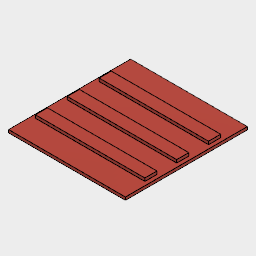
HDD Base Plate v5 (Autodesk Fusion 360 design; units mm, degrees)
Autodesk Fusion 360 part; units mm, degrees
sketch "Sketch1" plane through (0, 0, 0) normal (0, 1, 0) x (1, 0, 0) in component "HDD"
  line L0 (0, 0) -> (-146, 0)
  line L1 (-146, 0) -> (-146, 25.4)
  line L2 (-146, 25.4) -> (0, 25.4)
  line L3 (0, 25.4) -> (0, 0)
  dimension "d1" = 146
  dimension "d2" = 25.4
  measures "d1" distance of L0.start L0.end
  measures "d2" distance of L0.start L2.end
extrude "Extrude1" add sketch "Sketch1" along normal blind 101.6 makes body 1 in component "HDD"
sketch "Sketch1 (2)" plane through (0, 0, 0) normal (0, 1, 0) x (1, 0, 0) in component "Base"
  line L0 (0, 0) -> (-146, 0)
  line L1 (-146, 0) -> (-146, 153)
  line L2 (-146, 153) -> (0, 153)
  line L3 (0, 153) -> (0, 0)
  dimension "d8" = 153
  dimension "d9" = 146
  measures "d8" distance of L0.start L2.end
  measures "d9" distance of L0.start L0.end
extrude "Extrude1'" add sketch "Sketch1 (2)" along normal blind 4 separate body makes body 2 in component "Base"
pattern_linear "R-Pattern1" [suppressed]
extrude "Extrude2" add 1 faces at (-48.6667, 1.3333, 0) along direction (0, 0, 1) blind 5 on bodies 2 bodies 2 in component "Base"
extrude "Extrude3" add 1 faces at (0, 2.6667, -100.3333) along direction (1, 0, 0) blind 5 on bodies 2 bodies 2 in component "Base"
extrude "Extrude4" add 1 faces at (-95.6667, 1.3333, -153) along direction (0, 0, -1) blind 5 on bodies 2 bodies 2 in component "Base"
extrude "Extrude5" add 1 faces at (-146, 2.6667, -103.6667) along direction (-1, 0, 0) blind 5 on bodies 2 bodies 2 in component "Base"
sketch "Sketch1 (3)" plane through (0, 0, -127.6) normal (0, 0, 1) x (1, 0, 0)
  line L0 (-146, 0) -> (0, 0)
  line L1 (0, 0) -> (0, 101.6)
  line L2 (0, 101.6) -> (-146, 101.6)
  line L3 (-146, 101.6) -> (-146, 0)
sketch "Sketch2" plane through (0, 4, 0) normal (0, 1, 0) x (-1, 0, 0)
  line L0 (151, 5) -> (-5, 5)
  line L1 (-5, 5) -> (-5, -158)
  line L2 (-5, -158) -> (151, -158)
  line L3 (151, -158) -> (151, 5)
sketch "Sketch3" plane through (0, 0, 0) normal (0, 1, 0) x (1, 0, 0)
  line L0 (-146, 127.6) -> (0, 127.6)
  line L1 (0, 127.6) -> (0, 110.4667)
  line L2 (0, 110.4667) -> (-146, 110.4667)
  line L3 (-146, 110.4667) -> (-146, 127.6)
  point P0 (-146, 127.6)
  point P1 (0, 110.4667)
extrude "Extrude1''" add sketch "Sketch3" along normal blind 4 separate body makes body 3
move_body "Move1" bodies 3 to x (1, 0, 0) y (0, 1, 0) z (0, 0, 1) at (0, 35, 0)
extrude "Extrude2'" cut 1 faces at (-48.6667, 36.3333, -110.4667) along direction (0, 0, -1) blind 0.5 on bodies 3 bodies 3
extrude "Extrude3'" cut 1 faces at (-97.3333, 36.3333, -127.6) along direction (0, 0, 1) blind 0.5 on bodies 3 bodies 3
move_body "Align1" bodies 3 to x (1, 0, 0) y (0, 1, 0) z (0, 0, 1) at (0, -31, 0)
pattern_linear "R-Pattern1'" count 3 spacing 42.5 along (0, 0, 1) of bodies 3 makes body 4 at (-97.3333, 4, -79.2222) makes body 5 at (-97.3333, 4, -36.7222)
combine "Combine1" operation add target body 4 tool bodies 5 3 2
component "HDD" placed x (1, 0, 0) y (0, 1, 0) z (0, 0, 1) at (0, 0, 0)
component "Base" placed x (1, 0, 0) y (0, 1, 0) z (0, 0, 1) at (0, 0, 0)
component "HDD" placed x (1, 0, 0) y (0, 1, 0) z (0, 0, 1) at (0, 0, -42.5333)
component "HDD" placed x (1, 0, 0) y (0, 1, 0) z (0, 0, 1) at (0, 0, -85.0667)
component "HDD" placed x (1, 0, 0) y (0, 1, 0) z (0, 0, 1) at (0, 0, -127.6)
equation "d1 = hddLength"
equation "d2 = hddHeight"
equation "hddHeight = 25.4 mm"
equation "hddLength = 146 mm"
equation "hddWidth = 101.6 mm"
equation "d6 = hddWidth"
equation "d8 = baseLength"
equation "d9 = hddLength"
equation "hddSpacing = 20 mm"
equation "baseHeight = 4 mm"
equation "d12 = baseHeight"
equation "baseLength = 153 mm"
